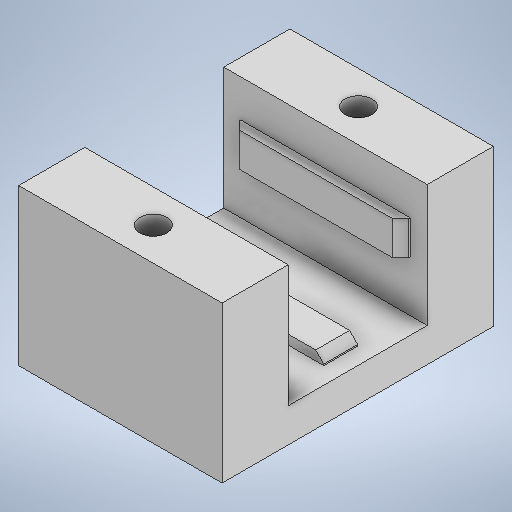
# Autodesk Inventor part: PingPongLauncherWinkel
Saved by Autodesk Inventor 2025 (Build 290162010, 162A)
## iProperties
Created: 2024-10-07
Part Number: PingPongLauncherWinkel
Material: Generisch
Document SubType Name: Modeling
Designer: max-h
Density: 1 g/cm^3
Appearance: Vorgabe
Author: max-h
Autodesk Inventor part; units mm, degrees
ref_plane "YZ Plane" through (0, 0, 0) normal (1, 0, 0) x (0, 1, 0)
ref_plane "XZ Plane" through (0, 0, 0) normal (0, 1, 0) x (-1, 0, 0)
ref_plane "XY Plane" through (0, 0, 0) normal (0, 0, 1) x (1, 0, 0)
sketch "Skizze16" plane through (0, 0, 0) normal (0, 1, 0) x (-1, 0, 0)
  line L0 (15, 20) -> (-15, 20)
  line L1 (-15, 20) -> (-15, -20)
  line L2 (-15, -20) -> (15, -20)
  line L3 (15, -20) -> (15, 20)
  line L4 (21, 0) -> (-21, 0) projected
  line L5 (0, -28) -> (0, 28) projected
  dimension "d82" = 40
  dimension "d83" = 30
  constraints: 8 end point, 2 parallel, 1 coincident, 1 horizontal, 1 perpendicular, 2 other
  measures "d82" distance between parallel lines of L2 L0
  measures "d83" distance of L0.start L0.end
extrude "Extrusion16" add sketch "Skizze16" along normal blind 5
sketch "Skizze17" plane through (0, 5, 0) normal (0, 1, 0) x (1, 0, 0)
  line L0 (-15, 20) -> (-15, -20) projected
  line L1 (15, -20) -> (15, 20) projected
  line L2 (-15, -20) -> (15, -20)
  line L3 (15, -20) -> (15, -10.25)
  line L4 (15, -10.25) -> (-15, -10.25)
  line L5 (-15, -10.25) -> (-15, -20)
  line L6 (-15, 20) -> (15, 20)
  line L7 (15, 20) -> (15, 10.25)
  line L8 (15, 10.25) -> (-15, 10.25)
  line L9 (-15, 10.25) -> (-15, 20)
  line L10 (-39, 0) -> (24, 0) projected
  dimension "d91" = 20.5
  constraints: 16 end point, 4 parallel, 3 point on line, 2 horizontal, 2 perpendicular, 1 other
  measures "d91" distance between parallel lines of L8 L4
extrude "Extrusion17" add sketch "Skizze17" along normal blind 18 contours L6 L1 L8 L0 | L4 L1 L2 L0
sketch "Skizze19" plane through (15, 5, 10.25) normal (0, 0, -1) x (-1, 0, 0)
  line L0 (2.5, 7.5) -> (27.5, 7.5)
  line L1 (27.5, 7.5) -> (27.5, 12.5)
  line L2 (27.5, 12.5) -> (2.5, 12.5)
  line L3 (2.5, 12.5) -> (2.5, 7.5)
  line L4 (30, 0) -> (0, 0) projected
  line L5 (0, 18) -> (30, 18) projected
  line L6 (15, 18) -> (15, 4.4527)
  line L7 (0, 0) -> (0, 18) projected
  point P0 (15, -5)
  dimension "d92" = 7.5
  dimension "d93" = 5
  dimension "d94" = 25
  dimension "d95" = 15
  constraints: 10 end point, 2 parallel, 1 horizontal, 1 midpoint, 1 perpendicular, 1 vertical, 1 other
  measures "d92" distance between parallel lines of L4 L0
  measures "d93" distance of L0.end L1.end
  measures "d94" distance between parallel lines of L1 L3
  measures "d95" distance between parallel lines of L7 L6
extrude "Extrusion18" add sketch "Skizze19" along normal blind 1.4
sketch "Skizze20" plane through (-15, 5, -10.25) normal (0, 0, 1) x (1, 0, 0)
  line L0 (2.5, 12.5) -> (27.5, 12.5) projected
  line L1 (27.5, 7.5) -> (2.5, 7.5) projected
  line L2 (2.5, 7.5) -> (2.5, 12.5) projected
  line L3 (27.5, 12.5) -> (27.5, 7.5) projected
  point P0 (15, -5)
extrude "Extrusion19" add sketch "Skizze20" along normal blind 1.4
sketch "Skizze21" plane through (0, 5, 0) normal (0, 1, 0) x (1, 0, 0)
  line L0 (-12.5, -2.5) -> (12.5, -2.5)
  line L1 (12.5, -2.5) -> (12.5, 2.5)
  line L2 (12.5, 2.5) -> (-12.5, 2.5)
  line L3 (-12.5, 2.5) -> (-12.5, -2.5)
  line L4 (-12.5, -10.25) -> (-12.5, -8.85) projected
  line L5 (12.5, -10.25) -> (12.5, -8.85) projected
  line L6 (-21, 0) -> (21, 0) projected
  point P0 (0, 0)
  dimension "d100" = 5
  constraints: 8 end point, 2 collinear, 2 parallel, 1 horizontal, 1 perpendicular, 1 other
  measures "d100" distance between parallel lines of L2 L0
extrude "Extrusion20" add sketch "Skizze21" along normal blind 1.4
chamfer "Fasen4" distance 1.2 angle 45 6 edges at (-12.5, 6.4, 0) (-12.5, 15, 8.85) (-12.5, 15, -8.85) (12.5, 15, 8.85) (12.5, 6.4, 0) (12.5, 15, -8.85)
sketch "Skizze22" plane through (0, 23, 0) normal (0, 1, 0) x (1, 0, 0)
  circle A0 centre (0, -15.125) radius 2
  circle A1 centre (0, 15.125) radius 2
  line L0 (0, 28) -> (0, -28) projected
  line L1 (-21, 0) -> (21, 0) projected
  line L2 (15, -10.25) -> (-15, -10.25) projected
  line L3 (-15, -20) -> (15, -20) projected
  point P0 (0, 0)
  dimension "d106" = 4
  dimension "d107" = 4.875
  constraints: 2 centre point, 2 point on line, 1 equal radius, 1 symmetric about line
  measures "d106" diameter of A0
  measures "d107" distance from line of L3 A0.centre
extrude "Extrusion21" cut sketch "Skizze22" against normal through all
chamfer "Fasen5" distance 2 angle 45 2 edges at (-2, 0, -15.125) (-2, 0, 15.125)
